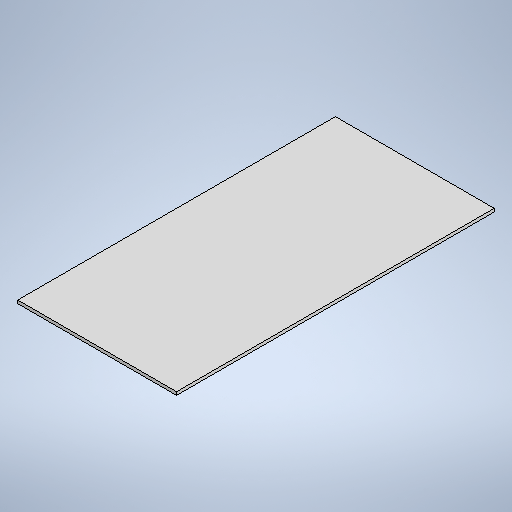
# Autodesk Inventor part: MSC 311 RIB BOARD
Saved by Autodesk Inventor 2025.1 (Build 291241020, 241B)
## iProperties
Created: 2024-04-28
Part Number: MSC 311 RIB BOARD
Material: Stainless Steel
Document SubType Name: Sheet Metal
Designer: admin
Density: 8 g/cm^3
Sheet Metal Rule: AISI304 2mm Die16
Appearance: Default
Sheet Metal Width: 0.000 mm
Sheet Metal Length: 0.000 mm
Sheet Metal Area: 0.000 mm^2
Stock Number: МОО 305 шпангоут борт
Description: DIE16(5)|\ 90°|corrY -___°|X_____|bom___
Mass: 1762.25 g
Surface Area: 2283.33 cm^2
Volume: 220.281 cm^3
БОРТ_стрингер_3_высота: 63.000 mm
БОРТ_стрингер_4_высота: 48.000 mm
БОРТ_стрингер_5_высота: 54.000 mm
БОРТ_стрингер_6_высота: 81.000 mm
РЕБРА_глубина_паза: 30,000 mm
РЕБРА_вырез_на_полке: 5,000 mm
РЕБРА_полка: 20,000 mm
Author: admin
Autodesk Inventor part; units mm, degrees
ref_plane "YZ Plane" through (0, 0, 0) normal (1, 0, 0) x (0, 1, 0)
ref_plane "XZ Plane" through (0, 0, 0) normal (0, 1, 0) x (-1, 0, 0)
ref_plane "XY Plane" through (0, 0, 0) normal (0, 0, 1) x (1, 0, 0)
sketch "Sketch1" plane through (0, 0, 0) normal (0, 0, 1) x (1, 0, 0)
  line L0 (-50, -100) -> (50, -100)
  line L1 (50, -100) -> (50, 100)
  line L2 (50, 100) -> (-50, 100)
  line L3 (-50, 100) -> (-50, -100)
  line L4 (-50, -100) -> (50, 100) construction
  line L5 (50, -100) -> (-50, 100) construction
  point P0 (0, 0)
  dimension "d154" = 100
  dimension "d155" = 200
  measures "d154" distance of L1.end L2.end
  measures "d155" distance of L0.end L1.end
extrude "Plate3" add sketch "Sketch1" along normal blind 2
equation "\"БОРТ_стрингер_3_высота\" = 63"
equation "\"БОРТ_стрингер_4_высота\" = 48"
equation "\"БОРТ_стрингер_5_высота\" = 54"
equation "\"БОРТ_стрингер_6_высота\" = 81"
body "Solid2"
